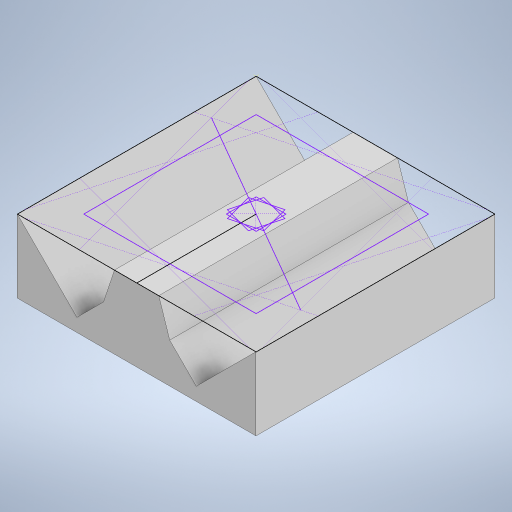
# Autodesk Inventor part: Drone Charging Base
Saved by Autodesk Inventor 2023 (Build 270158000, 158)
## iProperties
Created: 2022-12-15
Part Number: Drone Charging Base
Material: Generic
Document SubType Name: Modeling
Designer: chase
Density: 1 g/cm^3
Appearance: Default
Author: chase
Autodesk Inventor part; units mm, degrees
ref_plane "YZ Plane" through (0, 0, 0) normal (1, 0, 0) x (0, 1, 0)
ref_plane "XZ Plane" through (0, 0, 0) normal (0, 1, 0) x (-1, 0, 0)
ref_plane "XY Plane" through (0, 0, 0) normal (0, 0, 1) x (1, 0, 0)
sketch "Sketch1" plane through (0, 0, 0) normal (0, 0, 1) x (1, 0, 0)
  line L0 (0, 0) -> (914.4, 0)
  line L1 (914.4, 0) -> (914.4, 279.0857)
  line L2 (787.7143, 152.4) -> (126.6857, 152.4)
  line L3 (0, 279.0857) -> (0, 0)
  line L4 (457.2, 0) -> (457.2, 152.4)
  line L5 (685.8, 0) -> (685.8, 152.4)
  line L6 (228.6, 0) -> (228.6, 152.4)
  line L7 (228.6, 50.4857) -> (-130.6102, 409.6959)
  line L8 (228.6, 50.4857) -> (330.5143, 152.4)
  line L9 (685.8, 50.4857) -> (583.8857, 152.4)
  line L10 (685.8, 50.4857) -> (1045.0102, 409.6959)
  line L11 (330.2, 0) -> (330.2, 152.0857)
  line L12 (127, 0) -> (127, 152.4)
  line L13 (584.2, 0) -> (584.2, 152.0857)
  line L14 (787.4, 0) -> (787.4, 152.4)
  line L15 (372.331, 279.0857) -> (542.069, 279.0857)
  line L16 (372.331, 279.0857) -> (330.5143, 152.4)
  line L17 (542.069, 279.0857) -> (583.8857, 152.4)
  point P0 (330.2, 152.4)
  dimension "d18" = 101.6
  dimension "d19" = 101.6
  dimension "d20" = 101.6
  dimension "d21" = 101.6
  constraints: 34 end point, 9 point on line, 7 parallel, 3 horizontal, 1 midpoint, 1 perpendicular, 1 symmetric about line, 12 other
  measures "d18" distance between parallel lines of L6 L11
  measures "d19" distance between parallel lines of L6 L12
  measures "d20" distance between parallel lines of L5 L13
  measures "d21" distance between parallel lines of L5 L14
extrude "Extrusion1" add sketch "Sketch1" against normal blind 914.4 contours L3 L7 L12 L0 | L12 L7 L6 L0 | L6 L8 L11 L0 | L11 L8 L2 L4 L0 | L4 L2 L9 L13 L0 | L13 L9 L5 L0 | L2 L16 L15 L17 | L5 L10 L14 L0 | L14 L10 L1 L0
extrude "Extrusion2" add sketch "Sketch1" against normal blind 914.4 contours L2 L16 L15 L17
sketch "Sketch2" plane through (372.331, 279.0857, 0) normal (0, 1, 0) x (1, 0, 0)
  line L0 (169.738, 0) -> (0, 0) projected
  line L1 (84.869, 0) -> (84.869, 457.2)
  line L2 (-245.331, 787.4) -> (415.069, 787.4)
  line L3 (415.069, 787.4) -> (415.069, 127)
  line L4 (415.069, 127) -> (-245.331, 127)
  line L5 (-245.331, 127) -> (-245.331, 787.4)
  line L6 (27.719, 514.35) -> (142.019, 514.35)
  line L7 (142.019, 514.35) -> (142.019, 400.05)
  line L8 (142.019, 400.05) -> (27.719, 400.05)
  line L9 (27.719, 400.05) -> (27.719, 514.35)
  line L10 (27.719, 514.35) -> (142.019, 400.05) construction
  line L11 (142.019, 514.35) -> (27.719, 400.05) construction
  line L12 (-372.331, 676.5418) -> (515.3678, 914.4) construction
  line L13 (304.2108, 914.4) -> (542.069, 26.7012) construction
  line L14 (542.069, 237.8582) -> (-345.6298, 0) construction
  line L15 (-134.4728, 0) -> (-372.331, 887.6988) construction
  line L16 (-319.5418, 690.6867) -> (489.2797, 223.7133)
  line L17 (14.8748, 497.6112) -> (125.2801, 527.1942)
  line L18 (125.2801, 527.1942) -> (154.8631, 416.7888)
  line L19 (154.8631, 416.7888) -> (44.4578, 387.2058)
  line L20 (44.4578, 387.2058) -> (14.8748, 497.6112)
  line L21 (515.3678, 0) -> (-372.331, 237.8582) construction
  line L22 (-372.331, 26.7012) -> (-134.4728, 914.4) construction
  line L23 (-345.6298, 914.4) -> (542.069, 676.5418) construction
  line L24 (542.069, 887.6988) -> (304.2108, 0) construction
  line L25 (125.2801, 387.2058) -> (14.8748, 416.7888)
  line L26 (14.8748, 416.7888) -> (44.4578, 527.1942)
  line L27 (44.4578, 527.1942) -> (154.8631, 497.6112)
  line L28 (154.8631, 497.6112) -> (125.2801, 387.2058)
  line L29 (142.019, 514.35) -> (27.719, 400.05) construction
  line L30 (-372.331, 0) -> (542.069, 0) projected
  line L31 (-372.331, 914.4) -> (542.069, 914.4)
  line L32 (542.069, 914.4) -> (542.069, 0)
  line L33 (542.069, 0) -> (-372.331, 0)
  line L34 (-372.331, 0) -> (-372.331, 914.4)
  constraints: 66 end point, 20 point on line, 14 parallel, 7 perpendicular, 3 horizontal, 3 midpoint, 1 vertical
body "Solid1"
